Geschirrspueler_Stopfen_v1 (Autodesk Fusion 360 design; units mm, degrees)
Autodesk Fusion 360 part; units mm, degrees
sketch "Sketch1" plane through (0, 0, 0) normal (0, 1, 0) x (1, 0, 0)
  circle A0 centre (0, 0) radius 11
  circle A1 centre (0, 0) radius 7.5
  dimension "d1" = 22
  dimension "d2" = 15
  constraint coincident A0.centre A1.centre
  measures "d1" diameter of A0
  measures "d2" diameter of A1
ref_plane "WorkPlane1" through (0, 138, 0) normal (0, 1, 0) x (1, 0, 0)
ref_plane "WorkPlane2" through (0, -20, 0) normal (0, 1, 0) x (1, 0, 0)
sketch "Sketch2" plane through (0, -20, 0) normal (0, 1, 0) x (1, 0, 0)
  circle A0 centre (0, 0) radius 7.5
  circle A1 centre (0, 0) radius 10.5
  dimension "d5" = 21
  constraint concentric A0 A1
  measures "d5" diameter of A1
sketch "Sketch3" plane through (0, 138, 0) normal (0, 1, 0) x (1, 0, 0)
  circle A0 centre (0, 0) radius 7.5
  circle A1 centre (0, 0) radius 11
  line L0 (0, 0) -> (20, 0) construction
  line L1 (-12, 0) -> (13, 0)
  line L2 (-11.2763, -4.1042) -> (12.216, 4.4463)
  line L3 (-9.1925, -7.7135) -> (9.9586, 8.3562)
  line L4 (-6, -10.3923) -> (6.5, 11.2583)
  line L5 (-2.0838, -11.8177) -> (2.2574, 12.8025)
  line L6 (2.0838, -11.8177) -> (-2.2574, 12.8025)
  line L7 (6, -10.3923) -> (-6.5, 11.2583)
  line L8 (9.1925, -7.7135) -> (-9.9586, 8.3562)
  line L9 (11.2763, -4.1042) -> (-12.216, 4.4463)
  constraint horizontal L0
  constraint coincident A0.centre A1.centre
  constraint coincident L0 L1.end
  constraint parallel L0 L1
ref_plane "WorkPlane3" through (0, 148, 0) normal (0, 1, 0) x (1, 0, 0)
sketch "Sketch4" plane through (0, 148, 0) normal (0, 1, 0) x (1, 0, 0)
  circle A0 centre (0, 0) radius 7.5
  circle A1 centre (0, 0) radius 14
  dimension "d10" = 28
  constraint coincident A0.centre A1.centre
  measures "d10" diameter of A1
extrude "Extrude1" add sketch "Sketch4" along normal blind 2 contours A0 | A1 makes body 1
loft "Loft1" add profiles "Sketch2", "Sketch1", "Sketch3" section 1 section 2 section 3 contours A0 A1 L1 L9 | A0 A1 L1 L2 | A0 A1 L2 L3 | A0 A1 L8 L9 | A0 A1 L3 L4 | A0 A1 L7 L8 | A0 A1 L1 L9 | A0 A1 L1 L2 | A0 A1 L2 L3 | A0 A1 L3 L4 | A0 A1 L4 L5 | A0 A1 L4 L5 | A0 A1 L5 L6 | A0 A1 L5 L6 | A0 A1 L6 L7 | A0 A1 L6 L7 | A0 A1 L7 L8 | A0 A1 L8 L9 separate body makes body 2
extrude "Extrude2" cut sketch "Sketch2" along normal blind 160 contours A0 bodies 2
extrude "Extrude3" add sketch "Sketch3" along normal blind 10 contours A0 A1 L1 L9 | A0 A1 L2 L3 | A0 A1 L7 L8 | A0 A1 L1 L2 | A0 A1 L3 L4 | A0 A1 L4 L5 | A0 A1 L5 L6 | A0 A1 L6 L7 | A0 A1 L8 L9 picked at (9.446, -2.6762) picked at (9.0714, 3.7547) picked at (6.4214, -7.4266) picked at (-9.8085, -0.4257) picked at (-6.1987, -7.6135) picked at (2.1224, 9.5856) picked at (-0.1454, -9.8167) picked at (-4.5356, 8.7073) picked at (-9.0714, 3.7547) bodies 1 2
